Autodesk Inventor part; units mm, degrees
(part 2 of 2)
extrude "Extrusion1" add sketch "Sketch1" along normal blind 25 contours A0 | A1 A7 A6 A5 A2 A3 A4 | A8 A9 A10 A12 A11 A13 A1 | A1 A476 A477 A478 A480 A479 A481 | A14 A15 A16 A18 A17 A19 A1 | A1 A470 A471 A472 A474 A473 A475 | A20 A21 A22 A24 A23 A25 A1 | A1 A464 A465 A466 A468 A467 A469 | A26 A27 A28 A30 A29 A31 A1 | A1 A458 A459 A460 A462 A461 A463 | A32 A33 A34 A36 A35 A37 A1 | A1 A452 A453 A454 A456 A455 A457 | A38 A39 A40 A42 A41 A43 A1 | A1 A446 A447 A448 A450 A449 A451 | A44 A45 A46 A48 A47 A49 A1 | A1 A440 A441 A442 A444 A443 A445 | A50 A51 A52 A54 A53 A55 A1 | A1 A434 A435 A436 A438 A437 A439 | A56 A57 A58 A60 A59 A61 A1 | A1 A428 A429 A430 A432 A431 A433 | A62 A63 A64 A66 A65 A67 A1 | A1 A422 A423 A424 A426 A425 A427 | A68 A69 A70 A72 A71 A73 A1 | A1 A416 A417 A418 A420 A419 A421 | A74 A75 A76 A78 A77 A79 A1 | A1 A410 A411 A412 A414 A413 A415 | A80 A81 A82 A84 A83 A85 A1 | A1 A404 A405 A406 A408 A407 A409 | A86 A87 A88 A90 A89 A91 A1 | A1 A398 A399 A400 A402 A401 A403 | A92 A93 A94 A96 A95 A97 A1 | A1 A392 A393 A394 A396 A395 A397 | A98 A99 A100 A102 A101 A103 A1 | A1 A386 A387 A388 A390 A389 A391 | A104 A105 A106 A108 A107 A109 A1 | A1 A380 A381 A382 A384 A383 A385 | A110 A111 A112 A114 A113 A115 A1 | A1 A374 A375 A376 A378 A377 A379 | A116 A117 A118 A120 A119 A121 A1 | A1 A368 A369 A370 A372 A371 A373 | A122 A123 A124 A126 A125 A127 A1 | A1 A362 A363 A364 A366 A365 A367 | A128 A129 A130 A132 A131 A133 A1 | A1 A356 A357 A358 A360 A359 A361 | A134 A135 A136 A138 A137 A139 A1 | A1 A350 A351 A352 A354 A353 A355 | A140 A141 A142 A144 A143 A145 A1 | A1 A344 A345 A346 A348 A347 A349 | A146 A147 A148 A150 A149 A151 A1 | A1 A338 A339 A340 A342 A341 A343 | A152 A153 A154 A156 A155 A157 A1 | A1 A332 A333 A334 A336 A335 A337 | A158 A159 A160 A162 A161 A163 A1 | A1 A326 A327 A328 A330 A329 A331 | A164 A165 A166 A168 A167 A169 A1 | A1 A320 A321 A322 A324 A323 A325 | A170 A171 A172 A174 A173 A175 A1 | A1 A314 A315 A316 A318 A317 A319 | A176 A177 A178 A180 A179 A181 A1 | A1 A308 A309 A310 A312 A311 A313 | A182 A183 A184 A186 A185 A187 A1 | A1 A302 A303 A304 A306 A305 A307 | A188 A189 A190 A192 A191 A193 A1 | A1 A296 A297 A298 A300 A299 A301 | A194 A195 A196 A198 A197 A199 A1 | A1 A290 A291 A292 A294 A293 A295 | A200 A201 A202 A204 A203 A205 A1 | A1 A284 A285 A286 A288 A287 A289 | A206 A207 A208 A210 A209 A211 A1 | A1 A278 A279 A280 A282 A281 A283 | A212 A213 A214 A216 A215 A217 A1 | A1 A272 A273 A274 A276 A275 A277 | A218 A219 A220 A222 A221 A223 A1 | A1 A266 A267 A268 A270 A269 A271 | A224 A225 A226 A228 A227 A229 A1 | A1 A260 A261 A262 A264 A263 A265 | A230 A231 A232 A234 A233 A235 A1 | A1 A254 A255 A256 A258 A257 A259 | A236 A237 A238 A240 A239 A241 A1 | A1 A248 A249 A250 A252 A251 A253 | A242 A243 A244 A246 A245 A247 A1
equation "\"d9\" = GT2_R1"
equation "\"d10\" = GT2_R2"
equation "\"d11\" = GT2_R3"
equation "\"d12\" = GT2_H"
equation "\"d13\" = GT2_D"
equation "\"d18\" = THCK"
equation "\"GT2_R1\" = 0.15"
equation "\"GT2_R2\" = 1"
equation "\"GT2_R3\" = 0.555"
equation "\"GT2_D\" = 0.4"
equation "\"GT2_H\" = 0.75"
equation "\"THCK\" = 2 * parameter_extrusion_width"
equation "\"parameter_extrusion_width\" = 0.45"
equation "\"GT2_pitch\" = 2"
equation "\"parameter_belt_width\" = 25"
body "Solid1"
